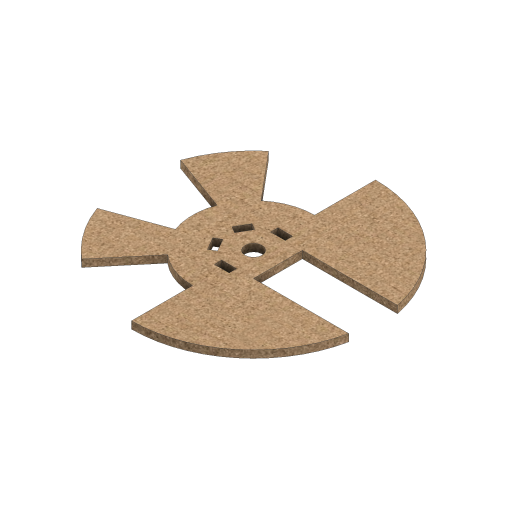
# Autodesk Inventor part: rolling_plate_small
Saved by Autodesk Inventor 2024 (Build 280153000, 153)
## iProperties
Created: 2024-04-09
Material: MDF Medium Density Fiberboard
Document SubType Name: Modeling
Designer: USER
Density: 0.8 g/cm^3
Appearance: Cardboard - Corrugated
Mass: 11.9681 g
Surface Area: 117.243 cm^2
Volume: 14.9601 cm^3
Author: 第26組
Title: rolling_plate_small
Autodesk Inventor part; units mm, degrees
ref_plane "YZ Plane" through (0, 0, 0) normal (1, 0, 0) x (0, 1, 0)
ref_plane "XZ Plane" through (0, 0, 0) normal (0, 1, 0) x (-1, 0, 0)
ref_plane "XY Plane" through (0, 0, 0) normal (0, 0, 1) x (1, 0, 0)
sketch "草圖1" plane through (0, 0, 0) normal (0, 1, 0) x (-1, 0, 0)
  circle A0 centre (0, 0) radius 50
  circle A1 centre (0, 0) radius 25
  line L0 (-50, 10) -> (-10, 10)
  line L1 (-10, 10) -> (-10, -10)
  line L2 (-10, -10) -> (-50, -10)
  line L3 (-50, -10) -> (-50, 10)
  line L4 (0, 0) -> (0, -50)
  line L5 (0, 0) -> (32.1394, -38.3022)
  arc A2 (0, -50) -> (32.1394, -38.3022) centre (0, 0) ccw
  line L6 (0, 0) -> (46.9846, -17.101)
  line L7 (0, 0) -> (46.9846, 17.101)
  arc A3 (46.9846, -17.101) -> (46.9846, 17.101) centre (0, 0) ccw
  line L8 (0, 0) -> (32.1394, 38.3022)
  line L9 (0, 0) -> (0, 50)
  arc A4 (32.1394, 38.3022) -> (0, 50) centre (0, 0) ccw
  circle A5 centre (0, 0) radius 3.5
  line L10 (-1.5, 3.1623) -> (-1.5, -3.1623)
  point P0 (16.0697, -19.1511)
  point P1 (0, -25)
  point P2 (-48.9898, 10)
  point P3 (-48.9898, -10)
  point P4 (16.0697, 19.1511)
  point P5 (0, 25)
  point P6 (23.4923, -8.5505)
  point P7 (23.4923, 8.5505)
  point P8 (-50, 0)
  dimension "d0" = 100
  dimension "d1" = 50
  dimension "d2" = 20
  dimension "d3" = 40
  dimension "d5" = 40
  dimension "d6" = 50
  dimension "d9" = 140
  dimension "d28" = 7
  dimension "d29" = 1.5
  dimension "d30" = 50
  constraints: 22 end point, 8 point on circle, 6 coincident, 5 centre point, 3 point on line, 2 parallel, 2 vertical, 1 horizontal, 1 horizontal alignment, 1 midpoint, 1 perpendicular, 20 other
  measures "d1" diameter of A1
  measures "d2" distance of L2.end L0.start
  measures "d3" distance of L1.end L2.end
  measures "d5" angle of L4 L5
  measures "d6" distance of L4.start L5.end
  measures "d28" diameter of A5
  measures "d29" distance between parallel lines of L4 L10
  measures "d30" radius of A2
extrude "擠出1" add sketch "草圖1" along normal blind 3 contours L7 A1 L8 A0 | A0 L5 A1 L6 | L7 A5 L8 A1 | A1 L6 A5 L7 | A1 L5 A5 L6 | L9 A1 L0 A0 | L8 A5 L9 A1 | A0 L2 A1 L4 | A1 L4 A5 L5 | L9 A5 L4 A1 L2 L1 L0
sketch "草圖2" plane through (0, 3, 0) normal (0, 1, 0) x (1, 0, 0)
  line L0 (-3, 13) -> (3, 13)
  line L1 (3, 13) -> (3, 10)
  line L2 (3, 10) -> (-3, 10)
  line L3 (-3, 10) -> (-3, 13)
  line L4 (-12.7583, 3.9019) -> (-9.7583, 9.0981)
  line L5 (-9.7583, 9.0981) -> (-7.1603, 7.5981)
  line L6 (-7.1603, 7.5981) -> (-10.1603, 2.4019)
  line L7 (-10.1603, 2.4019) -> (-12.7583, 3.9019)
  line L8 (-9.7583, -9.0981) -> (-12.7583, -3.9019)
  line L9 (-12.7583, -3.9019) -> (-10.1603, -2.4019)
  line L10 (-10.1603, -2.4019) -> (-7.1603, -7.5981)
  line L11 (-7.1603, -7.5981) -> (-9.7583, -9.0981)
  line L12 (3, -13) -> (-3, -13)
  line L13 (-3, -13) -> (-3, -10)
  line L14 (-3, -10) -> (3, -10)
  line L15 (3, -10) -> (3, -13)
  point P0 (0, 0)
  point P1 (0, 10)
  point P2 (-8.6603, 5)
  point P3 (-8.6603, -5)
  point P4 (0, -10)
  dimension "d31" = 3
  dimension "d32" = 6
  dimension "d33" = 10
  dimension "d36" = 180
  constraints: 32 end point, 2 parallel, 1 horizontal, 1 midpoint, 1 perpendicular, 1 vertical alignment, 28 other
  measures "d31" distance of L0.end L1.end
  measures "d32" distance of L1.end L2.end
  measures "d33" distance from line of point (0, 0) L2
extrude "擠出2" cut sketch "草圖2" against normal through all
